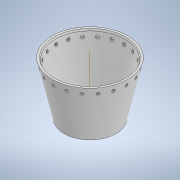
# Autodesk Inventor part: Box
Saved by Autodesk Inventor 2021 (Build 250183000, 183)
## iProperties
Created: 2021-04-16
Part Number: Box
Material: Generic
Document SubType Name: Modeling
Designer: tmass
Density: 1 g/cm^3
Appearance: Default
Author: tmass
Autodesk Inventor part; units mm, degrees
sketch "Sketch1" plane through (0, 0, 0) normal (0, 1, 0) x (-1, 0, 0)
  circle A0 centre (0, 0) radius 40.025
  dimension "d0" = 80.05
  constraints: 1 centre point, 1 coincident
  measures "d0" diameter of A0
ref_plane "Work Plane1" through (0, 90, 0) normal (0, 1, 0) x (-1, 0, 0)
sketch "Sketch2" plane through (0, 90, 0) normal (0, 1, 0) x (-1, 0, 0)
  circle A0 centre (0, 0) radius 60
  dimension "d4" = 120
  constraints: 1 centre point, 1 coincident
  measures "d4" diameter of A0
sketch "Sketch3" plane through (0, 0, 0) normal (1, 0, 0) x (0, 1, 0)
  line L0 (0, -44.025) -> (90.0381, -64)
  line L1 (90.0381, -64) -> (90.0381, -60)
  line L2 (90.0381, -60) -> (0, -40.025)
  line L3 (0, -40.025) -> (0, -44.025)
  line L4 (-18.0076, 0) -> (108.0457, 0) projected
  line L5 (0, 0) -> (0, -40.025)
  line L6 (90.0381, 0) -> (90.0381, -60)
  dimension "d6" = 4
  dimension "d17" = 40.025
  dimension "d18" = 60
  constraints: 12 end point, 4 vertical, 2 parallel, 1 point on line
  measures "d6" distance of L2.end L0.start
  measures "d17" distance of L2.end L5.start
  measures "d18" distance of L6.start L1.end
revolve "Revolution1" add sketch "Sketch3" angle 360 about axis through (0, -10, 0) along (0, 1, 0) contours L3 L2 L1 L0
ref_plane "Work Plane2" through (60, 0, 0) normal (1, 0, 0) x (0, 1, 0)
sketch "Sketch4" plane through (60, 0, 0) normal (1, 0, 0) x (0, 1, 0)
  circle A0 centre (80.0381, 0) radius 2.5
  line L0 (90.0381, 64) -> (90.0381, -64) projected
  point P0 (0, 0)
  dimension "d9" = 5
  dimension "d10" = 10
  constraints: 1 centre point
  measures "d9" diameter of A0
  measures "d10" distance from line of L0 A0.centre
extrude "Extrusion1" cut sketch "Sketch4" against normal mid plane 100
pattern_circular "Circular Pattern1" count 20 over 360 about axis through (0, -10, 0) along (0, 1, 0) of "Extrusion1"
chamfer "Chamfer1" distance 3 angle 10 1 edges at (0, 90.0381, 60) measured on face at (-4.1076, 40.8524, -48.916)
ref_plane "Work Plane3" through (0, 0, -65) normal (0, 0, 1) x (1, 0, 0)
body "Solid1"
